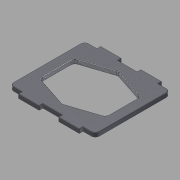
# Autodesk Inventor part: FPV Plate
Saved by Autodesk Inventor 2011 SP2 (Build 150309200, 309)
## iProperties
Created: 2015-02-19
Part Number: FPV Plate
Document SubType Name: Modeling
Designer: Greg Pavlik
Density: 1 g/cm^3
Author: Greg Pavlik
Autodesk Inventor part; units mm, degrees
ref_plane "YZ Plane" through (0, 0, 0) normal (1, 0, 0) x (0, 1, 0)
ref_plane "XZ Plane" through (0, 0, 0) normal (0, 1, 0) x (-1, 0, 0)
ref_plane "XY Plane" through (0, 0, 0) normal (0, 0, 1) x (1, 0, 0)
sketch "Sketch1" plane through (0, 0, 0) normal (0, 0, 1) x (1, 0, 0)
  line L0 (0, 17.5) -> (0, -17.5) construction
  line L1 (-20, 0) -> (20, 0) construction
  line L2 (20, 15.5) -> (20, -15.5)
  line L3 (-20, -15.5) -> (-20, 15.5)
  line L4 (-14.25, 19) -> (-4.5, 19)
  line L5 (-4.5, 19) -> (-4.5, 17.5)
  line L6 (-14.25, 17.5) -> (-14.25, 19)
  line L7 (4.5, 19) -> (14.25, 19)
  line L8 (14.25, 19) -> (14.25, 17.5)
  line L9 (4.5, 17.5) -> (4.5, 19)
  line L10 (4.5, -19) -> (14.25, -19)
  line L11 (14.25, -19) -> (14.25, -17.5)
  line L12 (4.5, -17.5) -> (4.5, -19)
  line L13 (-14.25, -19) -> (-4.5, -19)
  line L14 (-4.5, -19) -> (-4.5, -17.5)
  line L15 (-14.25, -17.5) -> (-14.25, -19)
  line L16 (14.25, 17.5) -> (18, 17.5)
  line L17 (-18, 17.5) -> (-14.25, 17.5)
  line L18 (-4.5, 17.5) -> (4.5, 17.5)
  line L19 (-14.25, -17.5) -> (-18, -17.5)
  line L20 (18, -17.5) -> (14.25, -17.5)
  line L21 (4.5, -17.5) -> (-4.5, -17.5)
  arc A0 (18, -17.5) -> (20, -15.5) centre (18, -15.5) ccw
  arc A1 (20, 15.5) -> (18, 17.5) centre (18, 15.5) ccw
  arc A2 (-18, 17.5) -> (-20, 15.5) centre (-18, 15.5) ccw
  arc A3 (-20, -15.5) -> (-18, -17.5) centre (-18, -15.5) ccw
  line L22 (-15.5, 6.5531) -> (-15.5, -6.5531)
  line L23 (15.5, 6.5531) -> (15.5, -6.5531)
  line L24 (14.1257, -8.4527) -> (0.6257, -12.8996)
  line L25 (-0.6257, -12.8996) -> (-14.1257, -8.4527)
  line L26 (-14.1257, 8.4527) -> (-0.6257, 12.8996)
  line L27 (0.6257, 12.8996) -> (14.1257, 8.4527)
  arc A4 (0.6257, 12.8996) -> (-0.6257, 12.8996) centre (0, 11) ccw
  arc A5 (15.5, 6.5531) -> (14.1257, 8.4527) centre (13.5, 6.5531) ccw
  arc A6 (14.1257, -8.4527) -> (15.5, -6.5531) centre (13.5, -6.5531) ccw
  arc A7 (-0.6257, -12.8996) -> (0.6257, -12.8996) centre (0, -11) ccw
  arc A8 (-15.5, -6.5531) -> (-14.1257, -8.4527) centre (-13.5, -6.5531) ccw
  arc A9 (-14.1257, 8.4527) -> (-15.5, 6.5531) centre (-13.5, 6.5531) ccw
  line L28 (14.1257, 8.4527) -> (15.5, 8) construction
  line L29 (15.5, 6.5531) -> (15.5, 8) construction
  point P0 (0, 0)
  point P1 (0, -13.1057)
  point P2 (0, 13.1057)
  dimension "d0" = 40
  dimension "d1" = 15.5
  dimension "d2" = 5.75
  dimension "d3" = 1.5
  dimension "d4" = 35
  dimension "d5" = 2
  dimension "d6" = 4.5
  dimension "d7" = 2
  dimension "d8" = 26
  dimension "d9" = 8
  constraints: 60 end point, 22 tangent, 20 point on circle, 15 parallel, 10 centre point, 9 perpendicular, 8 equal radius, 7 horizontal, 6 midpoint, 6 point on line, 3 collinear, 1 vertical, 20 other
  measures "d0" distance between parallel lines of L2 L3
  measures "d1" distance between parallel lines of L5 L3
  measures "d2" distance between parallel lines of L6 L3
  measures "d3" distance between parallel lines of L17 L4
  measures "d4" distance between parallel lines of L19 L17
  measures "d5" radius of A0
  measures "d6" distance between parallel lines of L3 L22
  measures "d7" radius of A4
  measures "d9" distance from line of L1 L28.end
extrude "Extrusion1" add sketch "Sketch1" along normal mid plane 2
chamfer "Chamfer1" distance 0.15 angle 45 24 edges at (7.3757, 10.6761, 1) (15.1204, 7.7254, 1) (15.5, 0, 1) (15.1204, -7.7254, 1) (7.3757, -10.6761, 1) (0, -13, 1) (-7.3757, -10.6761, 1) (-15.1204, -7.7254, 1) (-15.5, 0, 1) (-15.1204, 7.7254, 1) (-7.3757, 10.6761, 1) (0, 13, 1) (7.3757, 10.6761, -1) (0, 13, -1) (-7.3757, 10.6761, -1) (-15.1204, 7.7254, -1) (-15.5, 0, -1) (-15.1204, -7.7254, -1) (-7.3757, -10.6761, -1) (0, -13, -1) (7.3757, -10.6761, -1) (15.1204, -7.7254, -1) (15.5, 0, -1) (15.1204, 7.7254, -1)
chamfer "Chamfer2" distance 0.15 angle 45 56 edges at (20, 0, 1) (19.4142, -16.9142, 1) (16.125, -17.5, 1) (19.4142, 16.9142, 1) (16.125, 17.5, 1) (20, 0, -1) (19.4142, 16.9142, -1) (16.125, 17.5, -1) (19.4142, -16.9142, -1) (16.125, -17.5, -1) (-20, 0, 1) (-19.4142, 16.9142, 1) (-16.125, 17.5, 1) (-19.4142, -16.9142, 1) (-16.125, -17.5, 1) (-20, 0, -1) (-19.4142, -16.9142, -1) (-16.125, -17.5, -1) (-19.4142, 16.9142, -1) (-16.125, 17.5, -1) (0, -17.5, -1) (0, -17.5, 1) (0, 17.5, 1) (0, 17.5, -1) (-14.25, -18.25, 1) (-14.25, -18.25, -1) (-4.5, -18.25, 1) (-4.5, -18.25, -1) (4.5, -18.25, -1) (4.5, -18.25, 1) (14.25, -18.25, 1) (14.25, -18.25, -1) (14.25, 18.25, 1) (14.25, 18.25, -1) (-4.5, 18.25, 1) (-4.5, 18.25, -1) (-14.25, 18.25, -1) (-14.25, 18.25, 1) (9.375, 19, -1) (9.375, 19, 1) (14.25, 19, 0) (4.5, 19, 0) (4.5, 18.25, 1) (4.5, 18.25, -1) (-4.5, 19, 0) (-9.375, 19, 1) (-14.25, 19, 0) (-9.375, 19, -1) (-14.25, -19, 0) (-9.375, -19, 1) (-9.375, -19, -1) (4.5, -19, 0) (9.375, -19, -1) (9.375, -19, 1) (-4.5, -19, 0) (14.25, -19, 0)
body "Solid1"
